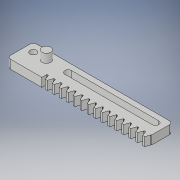
# Autodesk Inventor part: RackMirror
Saved by Autodesk Inventor 2019 (Build 230136000, 136)
## iProperties
Created: 2019-07-15
Part Number: RackMirror
Material: Generic
Document SubType Name: Modeling
Designer: aorfi
Density: 1 g/cm^3
Appearance: Default
Author: aorfi
Autodesk Inventor part; units mm, degrees
ref_plane "YZ Plane" through (0, 0, 0) normal (1, 0, 0) x (0, 1, 0)
ref_plane "XZ Plane" through (0, 0, 0) normal (0, 1, 0) x (-1, 0, 0)
ref_plane "XY Plane" through (0, 0, 0) normal (0, 0, 1) x (1, 0, 0)
sketch "Sketch1" plane through (0, 0, 0) normal (0, 1, 0) x (-1, 0, 0)
  line L0 (-40, 7.5) -> (40, 7.5)
  line L1 (40, 7.5) -> (40, -7.5)
  line L2 (40, -7.5) -> (-40, -7.5)
  line L3 (-40, -7.5) -> (-40, 7.5)
  line L4 (-40, 7.5) -> (40, -7.5) construction
  line L5 (40, 7.5) -> (-40, -7.5) construction
  circle A0 centre (15, -2.5) radius 1.8986
  circle A1 centre (-35, -2.5) radius 1.8986
  line L6 (15, -0.6014) -> (-35, -0.6014)
  line L7 (15, -4.3987) -> (-35, -4.3987)
  point P0 (0, 0)
  point P1 (0, 0)
  point P2 (35, 0)
  point P3 (0, 0)
  dimension "d0" = 80
  dimension "d1" = 15
  dimension "d8" = 5
  dimension "d61" = 3.7973
  dimension "d62" = 3.7973
  dimension "d63" = 5
  dimension "d64" = 5
  dimension "d65" = 50
  constraints: 16 end point, 4 midpoint, 4 point on circle, 3 tangent, 2 centre point, 2 horizontal, 2 horizontal alignment, 2 parallel, 1 perpendicular
  measures "d0" distance of L1.end L2.end
  measures "d1" distance of L0.end L1.end
  measures "d8" distance from line of L1 point (35, 0)
  measures "d61" diameter of A0
  measures "d62" diameter of A1
  measures "d63" distance from line of L2 A1.centre
  measures "d64" distance from line of A1.centre L3
  measures "d65" distance of L7.start L7.end
extrude "Extrusion1" add sketch "Sketch1" along normal mid plane 5
sketch "Sketch2" plane through (0, -2.5, 0) normal (0, -1, 0) x (1, 0, 0)
  line L0 (-40, 7.5) -> (-40, -7.5) projected
  line L1 (-40, -7.5) -> (40, -7.5) projected
  point P0 (0, 0)
  point P1 (-35, -2.5)
  point P2 (-40, 0)
  dimension "d16" = 5
  dimension "d60" = 5
  constraints: 1 midpoint
  measures "d16" distance from line of L0 point (-35, -2.5)
  measures "d60" distance from line of L1 point (-35, -2.5)
hole "Hole2" at (-35, -2.5, -2.5) direction (0, 1, 0) diameter 3.797 end through all clearance for "Flat Head Machine Screw (82)" size "#6" standard "Ansi Unified Screw Threads"
sketch "Sketch3" plane through (0, 2.5, 0) normal (0, -1, 0) x (1, 0, 0)
  circle A0 centre (-27.5, -2.5) radius 2.5
  line L0 (-40, 7.5) -> (-40, -7.5) projected
  circle A1 centre (-35, -2.5) radius 1.8985 projected
  point P0 (0, 0)
  point P1 (-40, 0)
  dimension "d24" = 5
  dimension "d26" = 7.5
  constraints: 1 centre point, 1 horizontal alignment, 1 midpoint
  measures "d24" diameter of A0
  measures "d26" distance of A0.centre A1.centre
extrude "Extrusion2" add sketch "Sketch3" against normal blind 5 contours A0
sketch "Sketch5" plane through (0, 2.5, 0) normal (0, -1, 0) x (1, 0, 0)
  arc A0 (35.771, 4.8227) -> (36.0102, 4.6552) centre (36.0102, 4.9098) ccw
  line L0 (36.0102, 4.6552) -> (36.5022, 4.6552)
  arc A1 (36.5022, 4.6552) -> (36.7414, 4.8227) centre (36.5022, 4.9098) ccw
  line L1 (36.7414, 4.8227) -> (37.7159, 7.5)
  line L2 (38.7863, 7.5) -> (37.7159, 7.5)
  line L3 (38.7863, 7.5) -> (39.7608, 4.8227)
  arc A2 (39.7608, 4.8227) -> (40, 4.6552) centre (40, 4.9098) ccw
  line L4 (36.5022, 4.9098) -> (40, 4.9098) construction
  line L5 (40, 7.5) -> (-40, 7.5) construction
  line L6 (40, -7.5) -> (40, 7.5) construction
  line L7 (35.771, 4.8227) -> (35.771, 10.6552)
  line L8 (35.771, 10.6552) -> (40, 10.6552)
  line L9 (40, 10.6552) -> (40, 4.6552)
  line L10 (40, -7.5) -> (-40, -7.5) projected
  dimension "d49" = 0.2546
  dimension "d50" = 0.2546
  dimension "d51" = 0.4921
  dimension "d52" = 1.0704
  dimension "d53" = 2.8448
  dimension "d54" = 3.0194
  dimension "d55" = 0.2546
  dimension "d68" = 15
  dimension "d69" = 6
  constraints: 16 end point, 6 point on circle, 4 tangent, 3 centre point, 3 horizontal alignment, 2 horizontal, 1 collinear, 1 perpendicular, 1 point on line, 1 vertical
  measures "d49" radius of A0
  measures "d50" radius of A1
  measures "d51" distance of L0.start L0.end
  measures "d52" distance of L2.start L1.end
  measures "d53" distance between parallel lines of L2 L0
  measures "d54" distance of L3.end L1.start
  measures "d55" radius of A2
  measures "d68" distance between parallel lines of L10 L2
  measures "d69" distance of L8.end L9.end
extrude "Extrusion4" cut sketch "Sketch5" along normal blind 5
pattern_linear "Rectangular Pattern1" count 15 spacing 3.99 along (-1, 0, 0) of "Extrusion4"
fillet "Fillet1" radius 2 3 edges at (-40, 0, 7.5) (-40, 0, -7.5) (40, 0, -7.5)
equation "\"d62\" = d61"
equation "\"d55\" = d50"
body "Solid1"
